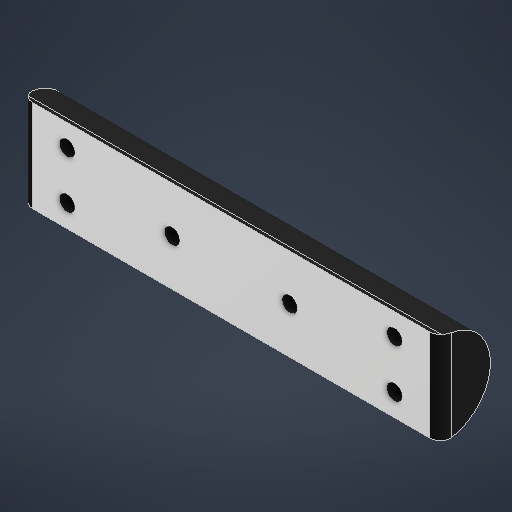
# Autodesk Inventor part: handle_insert
Saved by Autodesk Inventor 2026.1 (Build 301233000, 233)
## iProperties
Created: 2026-05-05
Part Number: handle_insert
Material: Generic
Document SubType Name: Modeling
Designer: aaron
Density: 1 g/cm^3
Appearance: Default
Author: aaron
Autodesk Inventor part; units mm, degrees
ref_plane "YZ Plane" through (0, 0, 0) normal (1, 0, 0) x (0, 1, 0)
ref_plane "XZ Plane" through (0, 0, 0) normal (0, 1, 0) x (-1, 0, 0)
ref_plane "XY Plane" through (0, 0, 0) normal (0, 0, 1) x (1, 0, 0)
sketch "Sketch1" plane through (0, 0, 0) normal (0, 0, 1) x (1, 0, 0)
  line L0 (0, 0) -> (114, 0)
  line L1 (114, 0) -> (114, 25)
  line L2 (114, 25) -> (0, 25)
  line L3 (0, 25) -> (0, 0)
  dimension "d0" = 25
  dimension "d1" = 114
  constraints: 8 end point, 2 parallel, 1 horizontal, 1 perpendicular
  measures "d0" distance of L2.end L0.start
  measures "d1" distance of L1.end L2.end
extrude "Extrusion1" add sketch "Sketch1" against normal blind 12.5
fillet "Fillet1" radius 12.5 2 edges at (57, 25, -12.5) (57, 0, -12.5)
sketch "Sketch2" plane through (0, 0, 0) normal (0, 0, 1) x (1, 0, 0)
  line L0 (114, 0) -> (114, 25) projected
  line L1 (114, 25) -> (0, 25) projected
  line L2 (0, 25) -> (0, 0) projected
  line L3 (0, 0) -> (114, 0) projected
extrude "Extrusion2" add sketch "Sketch2" along normal blind 1
fillet "Fillet2" radius 3 2 edges at (0, 12.5, 1) (114, 12.5, 1)
sketch "Sketch3" plane through (0, 0, 1) normal (0, 0, 1) x (1, 0, 0)
  circle A0 centre (12.38, 6) radius 1.6 projected
  circle A1 centre (12.38, 19) radius 1.6 projected
  circle A2 centre (40.88, 12.5) radius 1.6 projected
  circle A3 centre (72.88, 12.5) radius 1.6 projected
  circle A4 centre (101.38, 6) radius 1.6 projected
  circle A5 centre (101.38, 19) radius 1.6 projected
  circle A6 centre (12.38, 19) radius 2.15
  circle A7 centre (12.38, 6) radius 2.15
  circle A8 centre (40.88, 12.5) radius 2.15
  circle A9 centre (72.88, 12.5) radius 2.15
  circle A10 centre (101.38, 19) radius 2.15
  circle A11 centre (101.38, 6) radius 2.15
  point P0 (0, 0)
  dimension "d8" = 4.3
  dimension "d9" = 4.3
  dimension "d10" = 4.3
  dimension "d11" = 4.3
  dimension "d12" = 4.3
  dimension "d13" = 4.3
  constraints: 6 centre point, 6 coincident
  measures "d8" diameter of A6
  measures "d9" diameter of A7
  measures "d10" diameter of A8
  measures "d11" diameter of A9
  measures "d12" diameter of A10
  measures "d13" diameter of A11
extrude "Extrusion3" cut sketch "Sketch3" against normal blind 6 contours A0 | A1 | A2 | A3 | A4 | A5 | A6 | A7 | A8 | A9 | A10 | A11
equation "\"d9\" = d8"
equation "\"d10\" = d8"
equation "\"d11\" = d8"
equation "\"d12\" = d8"
equation "\"d13\" = d8"
body "Solid1"
